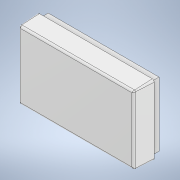
# Autodesk Inventor part: case_up
Saved by Autodesk Inventor 2022 (Build 260153000, 153)
## iProperties
Created: 2022-01-08
Part Number: case_up
Material: Пластик АБС
Document SubType Name: Modeling
Designer: Me
Density: 1.06 g/cm^3
Appearance: Гладкий — белый
Author: Me
Autodesk Inventor part; units mm, degrees
ref_plane "YZ Plane" through (0, 0, 0) normal (1, 0, 0) x (0, 1, 0)
ref_plane "XZ Plane" through (0, 0, 0) normal (0, 1, 0) x (-1, 0, 0)
ref_plane "XY Plane" through (0, 0, 0) normal (0, 0, 1) x (1, 0, 0)
sketch "Эскиз1" plane through (0, 0, 0) normal (0, 0, 1) x (1, 0, 0)
  line L0 (-29, 18) -> (29, 18)
  line L1 (30, 17) -> (30, -17)
  line L2 (29, -18) -> (-29, -18)
  line L3 (-30, -17) -> (-30, 17)
  arc A0 (-29, 18) -> (-30, 17) centre (-29, 17) ccw
  arc A1 (-30, -17) -> (-29, -18) centre (-29, -17) ccw
  arc A2 (29, -18) -> (30, -17) centre (29, -17) ccw
  arc A3 (30, 17) -> (29, 18) centre (29, 17) ccw
  point P0 (0, 0)
  point P1 (-30, 18)
  point P2 (30, 18)
  point P3 (-30, -18)
  dimension "d0" = 60
  dimension "d1" = 36
  dimension "d2" = 18
  dimension "d3" = 30
  dimension "d4" = 1
  constraints: 8 end point, 8 point on circle, 8 tangent, 6 point on line, 4 centre point, 3 equal radius, 2 parallel, 1 horizontal, 1 perpendicular
  measures "d0" distance of point (-30, 18) point (30, 18)
  measures "d1" distance of point (-30, -18) point (-30, 18)
  measures "d2" distance from line of point (0, 0) L0
  measures "d3" distance from line of point (0, 0) L1
  measures "d4" radius of A0
extrude "Выдавливание1" add sketch "Эскиз1" along normal blind 4
sketch "Эскиз3" plane through (0, 0, 4) normal (0, 0, 1) x (1, 0, 0)
  line L0 (-29, 18) -> (29, 18)
  line L1 (30, 17) -> (30, -17)
  line L2 (29, -18) -> (-29, -18)
  line L3 (-30, -17) -> (-30, 17)
  line L4 (30, -17) -> (30, 17) projected
  line L5 (-29, -18) -> (29, -18) projected
  line L6 (-30, 17) -> (-30, -17) projected
  line L7 (29, 18) -> (-29, 18) projected
  arc A0 (-29, 18) -> (-30, 17) centre (-29, 17) ccw
  arc A1 (-30, -17) -> (-29, -18) centre (-29, -17) ccw
  arc A2 (29, -18) -> (30, -17) centre (29, -17) ccw
  arc A3 (30, 17) -> (29, 18) centre (29, 17) ccw
  point P0 (0, 0)
  dimension "d7" = 0
  dimension "d8" = 0
  dimension "d9" = 0
  dimension "d10" = 0
  dimension "d11" = 1
  constraints: 8 end point, 8 point on circle, 8 tangent, 4 centre point, 3 equal radius, 2 parallel, 1 horizontal, 1 perpendicular
  measures "d7" distance between parallel lines of L4 L1
  measures "d8" distance between parallel lines of L5 L2
  measures "d9" distance between parallel lines of L6 L3
  measures "d10" distance between parallel lines of L7 L0
  measures "d11" radius of A0
extrude "Выдавливание2" add sketch "Эскиз3" along normal blind 10 draft -3
sketch "Эскиз4" plane through (0, 0, 0) normal (0, 0, -1) x (-1, 0, 0)
  line L0 (-27.5, 15.5) -> (27.5, 15.5)
  line L1 (27.5, 15.5) -> (27.5, -15.5)
  line L2 (27.5, -15.5) -> (-27.5, -15.5)
  line L3 (-27.5, -15.5) -> (-27.5, 15.5)
  point P0 (0, 0)
  dimension "d14" = 15.5
  dimension "d15" = 31
  dimension "d16" = 27.5
  dimension "d17" = 55
  constraints: 8 end point, 2 parallel, 1 horizontal, 1 perpendicular
  measures "d14" distance from line of point (0, 0) L0
  measures "d15" distance of L0.end L1.end
  measures "d16" distance from line of point (0, 0) L1
  measures "d17" distance of L0.start L0.end
extrude "Выдавливание3" cut sketch "Эскиз4" against normal blind 13 draft -3
sketch "Эскиз5" plane through (0, 0, 0) normal (0, 0, -1) x (-1, 0, 0)
  line L0 (-28.5, 16.5) -> (28.5, 16.5)
  line L1 (28.5, 16.5) -> (28.5, -16.5)
  line L2 (28.5, -16.5) -> (-28.5, -16.5)
  line L3 (-28.5, -16.5) -> (-28.5, 16.5)
  line L4 (-29, 18) -> (29, 18) projected
  line L5 (-30, -17) -> (-30, 17) projected
  line L6 (29, -18) -> (-29, -18) projected
  line L7 (30, 17) -> (30, -17) projected
  line L8 (-29, 18) -> (29, 18)
  line L9 (30, 17) -> (30, -17)
  line L10 (29, -18) -> (-29, -18)
  line L11 (-30, -17) -> (-30, 17)
  arc A0 (-29, 18) -> (-30, 17) centre (-29, 17) ccw
  arc A1 (-30, -17) -> (-29, -18) centre (-29, -17) ccw
  arc A2 (29, -18) -> (30, -17) centre (29, -17) ccw
  arc A3 (30, 17) -> (29, 18) centre (29, 17) ccw
  point P0 (0, 0)
  point P1 (29, 18)
  dimension "d20" = 1.5
  dimension "d21" = 1.5
  dimension "d22" = 1.5
  dimension "d23" = 1.5
  dimension "d24" = 0
  dimension "d25" = 0
  dimension "d26" = 0
  dimension "d27" = 0
  dimension "d28" = 1
  constraints: 16 end point, 8 point on circle, 8 tangent, 4 centre point, 4 parallel, 3 equal radius, 2 horizontal, 2 perpendicular
  measures "d20" distance between parallel lines of L4 L0
  measures "d21" distance between parallel lines of L5 L3
  measures "d22" distance between parallel lines of L6 L2
  measures "d23" distance between parallel lines of L7 L1
  measures "d24" distance between parallel lines of L4 L8
  measures "d25" distance between parallel lines of L5 L11
  measures "d26" distance between parallel lines of L6 L10
  measures "d27" distance between parallel lines of L7 L9
  measures "d28" radius of A0
extrude "Выдавливание4" cut sketch "Эскиз5" against normal blind 4
fillet "Сопряжение1" radius 1 8 edges at (-29.3365, -17.3365, 14) (-29.4759, 0, 14) (-29.3365, 17.3365, 14) (0, 17.4759, 14) (29.3365, 17.3365, 14) (29.4759, 0, 14) (29.3365, -17.3365, 14) (0, -17.4759, 14)
